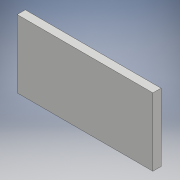
# Autodesk Inventor part: Phone
Saved by Autodesk Inventor 2017 (Build 210142000, 142)
## iProperties
Created: 2018-02-08
Part Number: Phone
Material: Generic
Document SubType Name: Modeling
Designer: Arjuna
Density: 1 g/cm^3
Appearance: Default
Author: Arjuna
Autodesk Inventor part; units mm, degrees
ref_plane "YZ Plane" through (0, 0, 0) normal (1, 0, 0) x (0, 1, 0)
ref_plane "XZ Plane" through (0, 0, 0) normal (0, 1, 0) x (-1, 0, 0)
ref_plane "XY Plane" through (0, 0, 0) normal (0, 0, 1) x (1, 0, 0)
sketch "Sketch1" plane through (0, 0, 0) normal (0, 1, 0) x (-1, 0, 0)
  line L0 (75, 37.5) -> (-75, 37.5)
  line L1 (-75, 37.5) -> (-75, -37.5)
  line L2 (-75, -37.5) -> (75, -37.5)
  line L3 (75, -37.5) -> (75, 37.5)
  point P0 (0, 0)
  dimension "d0" = 150
  dimension "d1" = 75
  dimension "d2" = 75
  dimension "d3" = 37.5
  constraints: 8 end point, 2 parallel, 1 horizontal, 1 perpendicular
  measures "d0" distance between parallel lines of L1 L3
  measures "d1" distance between parallel lines of L2 L0
  measures "d2" distance from line of point (0, 0) L3
  measures "d3" distance from line of point (0, 0) L0
extrude "Extrusion1" add sketch "Sketch1" along normal blind 9
sketch "Sketch3" plane through (0, 9, 0) normal (0, 1, 0) x (1, 0, 0)
  line L0 (-75, -37.5) -> (75, -37.5) projected
  line L1 (75, -37.5) -> (75, 37.5) projected
  line L2 (75, 37.5) -> (-75, 37.5) projected
  line L3 (-75, 37.5) -> (-75, -37.5) projected
  circle A0 centre (-44, 0) radius 12
  point P0 (0, 0)
  dimension "d11" = 24
  dimension "d12" = 19
  dimension "d13" = 31
  constraints: 1 centre point
  measures "d11" diameter of A0
  measures "d12" distance edge to line of A0 L3
  measures "d13" distance from line of A0.centre L3
extrude "Extrusion3" add sketch "Sketch3" along normal blind 2 contours A0
equation "\"d2\" = 0.5 * d0"
equation "\"d3\" = 0.5 * d1"
body "Solid1"
